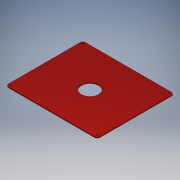
# Autodesk Inventor part: Structure_-ZCover
Saved by Autodesk Inventor 2018 (Build 220112000, 112)
## iProperties
Created: 2018-07-05
Part Number: Structure_-ZCover
Material: Aluminum 6061
Document SubType Name: Modeling
Designer: Bradley
Density: 2.7 g/cm^3
Appearance: Anodized - Red
Mass: 19.8306 g
Surface Area: 150.942 cm^2
Volume: 7.34467 cm^3
Author: Bradley
Autodesk Inventor part; units mm, degrees
ref_plane "YZ Plane" through (0, 0, 0) normal (1, 0, 0) x (0, 1, 0)
ref_plane "XZ Plane" through (0, 0, 0) normal (0, 1, 0) x (-1, 0, 0)
ref_plane "XY Plane" through (0, 0, 0) normal (0, 0, 1) x (1, 0, 0)
sketch "Sketch1" plane through (0, 0, 0) normal (0, 0, 1) x (1, 0, 0)
  line L0 (-45, -40) -> (45, -40)
  line L1 (47.5, -37.5) -> (47.5, 37.5)
  line L2 (45, 40) -> (-45, 40)
  line L3 (-47.5, 37.5) -> (-47.5, -37.5)
  line L4 (-47.5, -40) -> (47.5, 40) construction
  line L5 (47.5, -40) -> (-47.5, 40) construction
  arc A0 (-45, 40) -> (-47.5, 37.5) centre (-45, 37.5) ccw
  arc A1 (47.5, 37.5) -> (45, 40) centre (45, 37.5) ccw
  arc A2 (45, -40) -> (47.5, -37.5) centre (45, -37.5) ccw
  arc A3 (-47.5, -37.5) -> (-45, -40) centre (-45, -37.5) ccw
  point P0 (0, 0)
  dimension "d0" = 95
  dimension "d1" = 80
  dimension "d2" = 2.5
  constraints: 12 end point, 8 point on circle, 8 point on line, 8 tangent, 4 centre point, 3 equal radius, 2 midpoint, 2 parallel, 1 horizontal, 1 perpendicular
  measures "d0" distance of L4.end L5.end
  measures "d1" distance of L5.end L4.start
  measures "d2" radius of A0
extrude "Extrusion1" add sketch "Sketch1" along normal mid plane 1
sketch "Sketch2" plane through (0, 0, -0.5) normal (0, 0, -1) x (-1, 0, 0)
  circle A0 centre (0, 0) radius 9
  dimension "d5" = 18
  constraints: 1 centre point, 1 coincident
  measures "d5" diameter of A0
extrude "Extrusion2" cut sketch "Sketch2" against normal through all
sketch "Sketch3" plane through (0, 0, -0.5) normal (0, 0, -1) x (-1, 0, 0)
  circle A0 centre (0, 0) radius 9 projected
  line L0 (47.5, -37.5) -> (47.5, 37.5) projected
  arc A1 (47.5, 37.5) -> (45, 40) centre (45, 37.5) ccw projected
  line L1 (45, 40) -> (-45, 40) projected
  arc A2 (-45, 40) -> (-47.5, 37.5) centre (-45, 37.5) ccw projected
  line L2 (-47.5, 37.5) -> (-47.5, -37.5) projected
  arc A3 (-47.5, -37.5) -> (-45, -40) centre (-45, -37.5) ccw projected
  line L3 (-45, -40) -> (45, -40) projected
  arc A4 (45, -40) -> (47.5, -37.5) centre (45, -37.5) ccw projected
  constraints: 4 coincident
hole "Hole1" at (-45, -37.5, -0.5) at (45, -37.5, -0.5) at (45, 37.5, -0.5) at (-45, 37.5, -0.5) direction (0, 0, 1) diameter 2.2 end through all clearance for "Flat Head Machine Screw" size "M2" standard "Ansi Metric M Profile"
body "Solid1"
